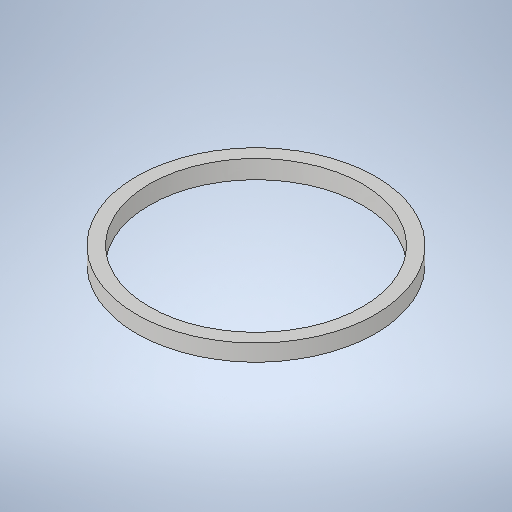
# Autodesk Inventor part: fenguangjinggai
Saved by Autodesk Inventor 2025.1 (Build 291241000, 241)
## iProperties
Created: 2024-08-22
Part Number: fenguangjinggai
Material: Generic
Document SubType Name: Sheet Metal
Designer: Administrator
Density: 1 g/cm^3
Sheet Metal Rule: 默认_mm
Appearance: Default
Author: Administrator
Autodesk Inventor part; units mm, degrees
ref_plane "YZ Plane" through (0, 0, 0) normal (1, 0, 0) x (0, 1, 0)
ref_plane "XZ Plane" through (0, 0, 0) normal (0, 1, 0) x (-1, 0, 0)
ref_plane "XY Plane" through (0, 0, 0) normal (0, 0, 1) x (1, 0, 0)
sketch "草图1" plane through (0, 0, 0) normal (0, 0, 1) x (1, 0, 0)
  line L0 (-12.2, 0) -> (-12.7, 0)
  line L1 (-12.7, 0) -> (-12.7, 1.6)
  line L2 (-12.7, 1.6) -> (-13.2, 1.6)
  line L3 (-13.2, 1.6) -> (-13.2, 0.2)
  line L4 (-13.2, 0.2) -> (-13.7, 0.2)
  line L5 (-13.7, 0.2) -> (-13.7, 1.6)
  line L6 (-13.7, 1.6) -> (-13.7, 2.1)
  line L7 (-13.7, 2.1) -> (-12.2, 2.1)
  line L8 (-12.2, 2.1) -> (-12.2, 0)
  line L9 (-12.2, 0) -> (-12.7, 0)
  line L10 (0, 0) -> (0.0001, 4.399)
  constraints: 22 end point, 7 perpendicular, 2 point on line, 1 horizontal
revolve "旋转1" add sketch "草图1" angle 360 about axis through (0, 0, 0) along (0, 1, 0)
equation "\"BendRadius\" = Thickness"
equation "\"BendReliefWidth\" = Thickness"
equation "\"BendReliefDepth\" = 0.5 * Thickness"
equation "\"CornerReliefSize\" = 4 * Thickness"
equation "\"MinimumRemnant\" = 2 * Thickness"
equation "\"TransitionRadius\" = BendRadius"
equation "\"JacobiRadiusSize\" = BendRadius"
equation "\"GapSize\" = Thickness"
equation "\"Thickness\" = 0.5"
